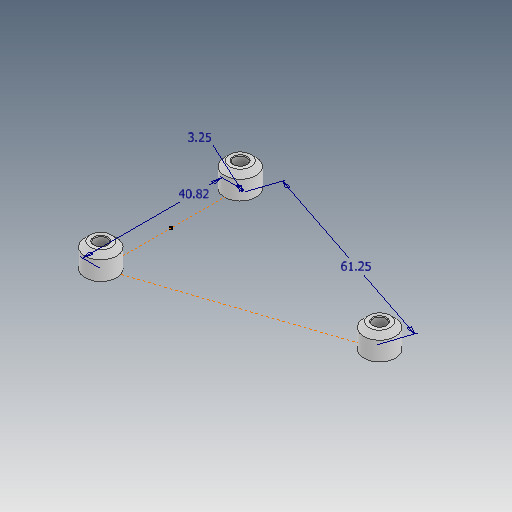
# Autodesk Inventor part: db-25_standoffs
Saved by Autodesk Inventor 2025.1 (Build 291241000, 241)
## iProperties
Created: 2026-06-20
Part Number: db-25_standoffs
Material: Generic
Document SubType Name: Modeling
Designer: Aiden
Density: 1 g/cm^3
Appearance: Default
Author: Aiden
Autodesk Inventor part; units mm, degrees
ref_plane "YZ Plane" through (0, 0, 0) normal (1, 0, 0) x (0, 1, 0)
ref_plane "XZ Plane" through (0, 0, 0) normal (0, 1, 0) x (-1, 0, 0)
ref_plane "XY Plane" through (0, 0, 0) normal (0, 0, 1) x (1, 0, 0)
sketch "Sketch1" plane through (0, 0, 0) normal (0, 1, 0) x (-1, 0, 0)
  circle A0 centre (42.9488, 7.9638) radius 1.625 construction
  circle A1 centre (-18.2369, 28.3738) radius 1.625 construction
  circle A2 centre (42.9488, 48.7838) radius 1.625 construction
  line L0 (42.9488, 7.9638) -> (42.9488, 48.7838) construction
  line L1 (41.4073, 48.2696) -> (-16.6954, 28.888) construction
  point P0 (42.9488, 28.3738)
  dimension "d0" = 3.25
  dimension "d22" = 40.82
  dimension "d23" = 61.25
  constraints: 4 end point, 1 centre point, 1 horizontal alignment, 1 midpoint, 1 vertical, 1 vertical alignment, 10 other
  measures "d0" diameter of A0
  measures "d22" distance of L0.start L0.end
sketch "Sketch2" plane through (0, 0, 0) normal (0, 1, 0) x (-1, 0, 0)
  circle A0 centre (42.9488, 7.9638) radius 1.625 construction
  circle A1 centre (-18.2369, 28.3738) radius 1.625 construction
  circle A2 centre (-38.2801, 41.1042) radius 1.6 construction
  circle A3 centre (42.9488, 48.7838) radius 1.625 construction
  circle A4 centre (42.9488, 7.9638) radius 3.625
  circle A5 centre (-18.2369, 28.3738) radius 3.625
  circle A6 centre (-38.2801, 41.1042) radius 3.625
  circle A7 centre (42.9488, 48.7838) radius 3.625
  point P0 (0, 0)
  dimension "d6" = 2
  constraints: 4 centre point, 4 coincident, 3 equal radius
  measures "d6" radial gap between concentric circles of A0 A4
extrude "Extrusion1" add sketch "Sketch2" along normal blind 7 contours A4 | A5 | A7
sketch "Sketch3" plane through (-42.9488, 7, 7.9638) normal (0, 1, 0) x (1, 0, 0)
  circle A0 centre (0, 0) radius 3.625 projected
  circle A1 centre (61.1856, -20.41) radius 3.625 projected
  circle A2 centre (0, -40.82) radius 3.625 projected
  point P0 (42.9488, 7.9638)
  point P1 (81.2288, -33.1404)
  point P2 (81.2288, -33.1404)
  constraints: 4 coincident
hole "Hole1" at (-42.9488, 7, 7.9638) at (18.2369, 7, 28.3738) at (38.2801, 7, 41.1042) at (-42.9488, 7, 48.7838) direction (0, -1, 0) diameter 3.75 end through all
chamfer "Chamfer1" distance 0.2 angle 45 3 edges at (-42.9488, 7, 6.0888) (18.2369, 7, 26.4988) (-42.9488, 7, 46.9088)
thicken "Thicken1" operation add thickness 1 both sides no extend neighbours no toward (-0.9870503, 0, -0.1604113) faces at (-46.5268, 4.6667, 7.3823)
thicken "Thicken2" operation add thickness 1 both sides no extend neighbours no toward (-0.9870503, 0, -0.1604113) faces at (-46.5268, 4.6667, 48.2023)
thicken "Thicken3" operation add thickness 1 both sides no extend neighbours no toward (-0.9870503, 0, -0.1604113) faces at (14.6588, 4.6667, 27.7923)
chamfer "Chamfer2" distance 1.5 angle 45 3 edges at (-38.3238, 7, 7.9638) (-38.3238, 7, 48.7838) (22.8619, 7, 28.3738)
body "Solid1"
